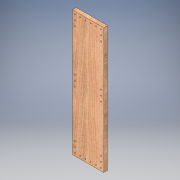
# Autodesk Inventor part: Side Board
Saved by Autodesk Inventor 2018 (Build 220112000, 112)
## iProperties
Created: 2018-12-30
Part Number: Side Board
Material: Generic
Document SubType Name: Modeling
Designer: maste
Density: 1 g/cm^3
Appearance: Default
Author: maste
Autodesk Inventor part; units mm, degrees
ref_plane "YZ Plane" through (0, 0, 0) normal (1, 0, 0) x (0, 1, 0)
ref_plane "XZ Plane" through (0, 0, 0) normal (0, 1, 0) x (-1, 0, 0)
ref_plane "XY Plane" through (0, 0, 0) normal (0, 0, 1) x (1, 0, 0)
sketch "Sketch1" plane through (0, 0, 0) normal (0, 0, 1) x (1, 0, 0)
  line L0 (0, 0) -> (152.4, 0)
  line L1 (152.4, 0) -> (152.4, 609.6)
  line L2 (152.4, 609.6) -> (0, 609.6)
  line L3 (0, 609.6) -> (0, 0)
  dimension "d0" = 152.4
  dimension "d1" = 609.6
  constraints: 8 end point, 2 parallel, 1 horizontal, 1 perpendicular
  measures "d0" distance of L2.end L1.end
  measures "d1" distance of L1.end L0.end
extrude "Extrusion1" add sketch "Sketch1" along normal blind 19.05
sketch "Sketch2" plane through (0, 0, 19.05) normal (0, 0, 1) x (1, 0, 0)
  line L0 (152.4, 609.6) -> (0, 609.6) construction
  line L1 (0, 609.6) -> (12.7, 609.6) construction
  line L2 (12.7, 609.6) -> (12.7, 596.9) construction
  line L3 (76.2, 609.6) -> (76.2, 0) construction
  line L4 (0, 0) -> (152.4, 0) construction
  line L5 (0, 609.6) -> (0, 0) construction
  line L6 (0, 304.8) -> (152.4, 304.8) construction
  line L7 (152.4, 0) -> (152.4, 609.6) construction
  circle A0 centre (12.7, 596.9) radius 2.5797
  circle A1 centre (139.7, 596.9) radius 2.5797
  circle A2 centre (12.7, 12.7) radius 2.5797
  circle A3 centre (139.7, 12.7) radius 2.5797
  dimension "d4" = 12.7
  dimension "d5" = 12.7
  dimension "d6" = 5.1594
  constraints: 8 end point, 4 centre point, 4 midpoint, 3 symmetric about line, 1 coincident, 1 perpendicular, 1 point on line, 3 other
  measures "d4" distance of L0.end L1.end
  measures "d5" distance of L1.end L2.end
  measures "d6" diameter of A0
extrude "Extrusion2" cut sketch "Sketch2" against normal blind 19.05
sketch "Sketch3" plane through (0, 0, 19.05) normal (0, 0, 1) x (1, 0, 0)
  circle A0 centre (12.7, 12.7) radius 2.5797 construction
  line L0 (12.7, 12.7) -> (12.7, 38.1) construction
  line L1 (12.7, 38.1) -> (12.7, 63.5) construction
  line L2 (12.7, 12.7) -> (38.1, 12.7) construction
  line L3 (38.1, 12.7) -> (63.5, 12.7) construction
  circle A1 centre (38.1, 12.7) radius 2.5797
  circle A2 centre (63.5, 12.7) radius 2.5797
  circle A3 centre (12.7, 38.1) radius 2.5797
  circle A4 centre (12.7, 63.5) radius 2.5797
  line L4 (0, 0) -> (152.4, 0) construction
  line L5 (76.2, 0) -> (76.2, 609.6) construction
  line L6 (0, 609.6) -> (0, 0) construction
  line L7 (0, 304.8) -> (152.4, 304.8) construction
  circle A5 centre (139.7, 12.7) radius 2.5797 construction
  line L8 (139.7, 12.7) -> (139.7, 38.1) construction
  line L9 (139.7, 38.1) -> (139.7, 63.5) construction
  line L10 (139.7, 12.7) -> (114.3, 12.7) construction
  line L11 (114.3, 12.7) -> (88.9, 12.7) construction
  circle A6 centre (114.3, 12.7) radius 2.5797
  circle A7 centre (88.9, 12.7) radius 2.5797
  circle A8 centre (139.7, 38.1) radius 2.5797
  circle A9 centre (139.7, 63.5) radius 2.5797
  line L12 (152.4, 0) -> (0, 0) construction
  line L13 (152.4, 609.6) -> (152.4, 0) construction
  circle A10 centre (12.7, 596.9) radius 2.5797 construction
  line L14 (12.7, 596.9) -> (12.7, 571.5) construction
  line L15 (12.7, 571.5) -> (12.7, 546.1) construction
  line L16 (12.7, 596.9) -> (38.1, 596.9) construction
  line L17 (38.1, 596.9) -> (63.5, 596.9) construction
  circle A11 centre (38.1, 596.9) radius 2.5797
  circle A12 centre (63.5, 596.9) radius 2.5797
  circle A13 centre (12.7, 571.5) radius 2.5797
  circle A14 centre (12.7, 546.1) radius 2.5797
  line L18 (0, 609.6) -> (152.4, 609.6) construction
  line L19 (76.2, 609.6) -> (76.2, 0) construction
  line L20 (0, 0) -> (0, 609.6) construction
  circle A15 centre (139.7, 546.1) radius 2.5797
  line L21 (139.7, 571.5) -> (139.7, 546.1) construction
  circle A16 centre (139.7, 571.5) radius 2.5797
  line L22 (139.7, 596.9) -> (139.7, 571.5) construction
  line L23 (139.7, 596.9) -> (114.3, 596.9) construction
  line L24 (114.3, 596.9) -> (88.9, 596.9) construction
  circle A17 centre (139.7, 596.9) radius 2.5797 construction
  circle A18 centre (114.3, 596.9) radius 2.5797
  circle A19 centre (88.9, 596.9) radius 2.5797
  line L25 (152.4, 609.6) -> (0, 609.6) construction
  line L26 (152.4, 0) -> (152.4, 609.6) construction
  dimension "d9" = 25.4
  dimension "d10" = 25.4
  dimension "d11" = 25.4
  dimension "d12" = 25.4
  constraints: 50 end point, 38 symmetric about line, 19 centre point, 16 coincident, 8 point on line, 2 horizontal, 2 midpoint, 2 vertical, 15 other
  measures "d9" distance of L0.start L0.end
  measures "d10" distance of L0.end L1.end
  measures "d11" distance of L0.start L2.end
  measures "d12" distance of L2.end L3.end
extrude "Extrusion3" cut sketch "Sketch3" against normal blind 19.05
sketch "Sketch4" plane through (0, 0, 19.05) normal (0, 0, 1) x (1, 0, 0)
  line L0 (152.4, 609.6) -> (0, 609.6) construction
  line L1 (76.2, 609.6) -> (76.2, 0) construction
  line L2 (152.4, 609.6) -> (152.4, 317.5) construction
  line L3 (152.4, 0) -> (152.4, 609.6) construction
  line L4 (152.4, 317.5) -> (152.4, 304.8) construction
  line L5 (152.4, 317.5) -> (139.7, 317.5) construction
  circle A0 centre (139.7, 317.5) radius 2.5797
  line L6 (139.7, 317.5) -> (139.7, 342.9) construction
  line L7 (139.7, 342.9) -> (139.7, 292.1) construction
  circle A1 centre (139.7, 342.9) radius 2.5797
  circle A2 centre (139.7, 292.1) radius 2.5797
  line L8 (0, 317.5) -> (12.7, 317.5) construction
  circle A3 centre (12.7, 317.5) radius 2.5797
  line L9 (12.7, 317.5) -> (12.7, 342.9) construction
  line L10 (12.7, 342.9) -> (12.7, 292.1) construction
  circle A4 centre (12.7, 342.9) radius 2.5797
  circle A5 centre (12.7, 292.1) radius 2.5797
  point P0 (0, 0)
  dimension "d15" = 292.1
  dimension "d17" = 12.7
  dimension "d19" = 5.1594
  dimension "d22" = 25.4
  dimension "d23" = 50.8
  constraints: 18 end point, 7 symmetric about line, 6 centre point, 6 coincident, 3 point on line, 2 midpoint, 2 vertical, 1 horizontal, 3 other
  measures "d15" distance of L0.start L2.end
  measures "d17" distance of L2.end L5.end
  measures "d19" diameter of A0
  measures "d22" distance of L6.start L6.end
  measures "d23" distance of L6.end L7.end
extrude "Extrusion5" cut sketch "Sketch4" against normal blind 19.05
body "Solid1"
